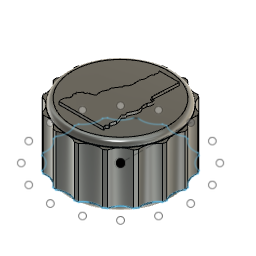
crown v4 (Autodesk Fusion 360 design; units mm, degrees)
Autodesk Fusion 360 part; units mm, degrees
note: some values were not read from the file. Set by a fixed rule: which sketch regions a step uses.
sketch "Sketch1" plane through (0, 0, 0) normal (0, 0, 1) x (1, 0, 0)
  line L0 (0, 0) -> (0, 2.54) construction
  line L1 (0, 2.54) -> (0, 3.1814)
  arc A0 (0.5741, 2.4743) -> (1.3436, 2.1555) centre (1.2174, 2.9392) ccw
  arc A1 (1.4773, 2.0662) -> (2.0662, 1.4773) centre (2.2496, 2.2496) ccw
  arc A2 (2.1555, 1.3436) -> (2.4743, 0.5741) centre (2.9392, 1.2174) ccw
  arc A3 (2.5056, 0.4165) -> (2.5056, -0.4165) centre (3.1814, 0) ccw
  arc A4 (2.4743, -0.5741) -> (2.1555, -1.3436) centre (2.9392, -1.2174) ccw
  arc A5 (2.0662, -1.4773) -> (1.4773, -2.0662) centre (2.2496, -2.2496) ccw
  arc A6 (1.3436, -2.1555) -> (0.5741, -2.4743) centre (1.2174, -2.9392) ccw
  arc A7 (-1.3436, 2.1555) -> (-0.5741, 2.4743) centre (-1.2174, 2.9392) ccw
  arc A8 (-0.4165, 2.5056) -> (0.4165, 2.5056) centre (0, 3.1814) ccw
  arc A9 (-2.0662, 1.4773) -> (-1.4773, 2.0662) centre (-2.2496, 2.2496) ccw
  arc A10 (-2.4743, 0.5741) -> (-2.1555, 1.3436) centre (-2.9392, 1.2174) ccw
  arc A11 (-2.5056, -0.4165) -> (-2.5056, 0.4165) centre (-3.1814, 0) ccw
  arc A12 (-1.4773, -2.0662) -> (-2.0662, -1.4773) centre (-2.2496, -2.2496) ccw
  arc A13 (-2.1555, -1.3436) -> (-2.4743, -0.5741) centre (-2.9392, -1.2174) ccw
  arc A14 (-0.5741, -2.4743) -> (-1.3436, -2.1555) centre (-1.2174, -2.9392) ccw
  arc A15 (0.4165, -2.5056) -> (-0.4165, -2.5056) centre (0, -3.1814) ccw
  arc A16 (-1.3436, 2.1555) -> (-1.4773, 2.0662) centre (0, 0) ccw
  arc A17 (-2.0662, 1.4773) -> (-2.1555, 1.3436) centre (0, 0) ccw
  arc A18 (-2.4743, 0.5741) -> (-2.5056, 0.4165) centre (0, 0) ccw
  arc A19 (-2.5056, -0.4165) -> (-2.4743, -0.5741) centre (0, 0) ccw
  arc A20 (-2.1555, -1.3436) -> (-2.0662, -1.4773) centre (0, 0) ccw
  arc A21 (-1.4773, -2.0662) -> (-1.3436, -2.1555) centre (0, 0) ccw
  arc A22 (-0.5741, -2.4743) -> (-0.4165, -2.5056) centre (0, 0) ccw
  arc A23 (0.4165, -2.5056) -> (0.5741, -2.4743) centre (0, 0) ccw
  arc A24 (1.3436, -2.1555) -> (1.4773, -2.0662) centre (0, 0) ccw
  arc A25 (2.0662, -1.4773) -> (2.1555, -1.3436) centre (0, 0) ccw
  arc A26 (-0.4165, 2.5056) -> (-0.5741, 2.4743) centre (0, 0) ccw
  arc A27 (0.5741, 2.4743) -> (0.4165, 2.5056) centre (0, 0) ccw
  arc A28 (1.4773, 2.0662) -> (1.3436, 2.1555) centre (0, 0) ccw
  arc A29 (2.1555, 1.3436) -> (2.0662, 1.4773) centre (0, 0) ccw
  arc A30 (2.4743, -0.5741) -> (2.5056, -0.4165) centre (0, 0) ccw
  arc A31 (2.5056, 0.4165) -> (2.4743, 0.5741) centre (0, 0) ccw
  dimension "d1" = 5.08
  dimension "d3" = 0.6413
  constraint coincident L0.start A16.centre
  constraint coincident L0.end A16
  constraint vertical L0
  constraint parallel L0 L1
  constraint coincident A8.start A16
  constraint concentric A16 A17
  constraint concentric A17 A18
  constraint concentric A18 A19
  constraint concentric A19 A20
  constraint concentric A20 A21
  constraint concentric A21 A22
  constraint concentric A22 A23
  constraint concentric A23 A24
  constraint concentric A24 A25
  constraint concentric A25 A30
  constraint coincident A0.start A30
  constraint concentric A26 A30
  constraint concentric A27 A30
  constraint concentric A28 A30
  constraint concentric A29 A30
  constraint concentric A30 A31
  measures "d1" diameter of A16
  measures "d3" distance of L0.end L1.end
extrude "Extrude1" add sketch "Sketch1" along normal blind 2.286
sketch "Sketch2" plane through (0, 0, 2.286) normal (0, 0, 1) x (-1, 0, 0)
  arc A0 (-0.5741, -2.4743) -> (-0.4165, -2.5056) centre (0, 0) ccw
  arc A1 (0.4165, -2.5056) -> (-0.4165, -2.5056) centre (0, -3.1814) ccw
  arc A2 (0.4165, -2.5056) -> (0.5741, -2.4743) centre (0, 0) ccw
  arc A3 (1.3436, -2.1555) -> (0.5741, -2.4743) centre (1.2174, -2.9392) ccw
  arc A4 (1.3436, -2.1555) -> (1.4773, -2.0662) centre (0, 0) ccw
  arc A5 (2.0662, -1.4773) -> (1.4773, -2.0662) centre (2.2496, -2.2496) ccw
  arc A6 (2.0662, -1.4773) -> (2.1555, -1.3436) centre (0, 0) ccw
  arc A7 (2.4743, -0.5741) -> (2.1555, -1.3436) centre (2.9392, -1.2174) ccw
  arc A8 (2.4743, -0.5741) -> (2.5056, -0.4165) centre (0, 0) ccw
  arc A9 (2.5056, 0.4165) -> (2.5056, -0.4165) centre (3.1814, 0) ccw
  arc A10 (2.5056, 0.4165) -> (2.4743, 0.5741) centre (0, 0) ccw
  arc A11 (2.1555, 1.3436) -> (2.4743, 0.5741) centre (2.9392, 1.2174) ccw
  arc A12 (2.1555, 1.3436) -> (2.0662, 1.4773) centre (0, 0) ccw
  arc A13 (1.4773, 2.0662) -> (2.0662, 1.4773) centre (2.2496, 2.2496) ccw
  arc A14 (1.4773, 2.0662) -> (1.3436, 2.1555) centre (0, 0) ccw
  arc A15 (0.5741, 2.4743) -> (1.3436, 2.1555) centre (1.2174, 2.9392) ccw
  arc A16 (0.5741, 2.4743) -> (0.4165, 2.5056) centre (0, 0) ccw
  arc A17 (-0.4165, 2.5056) -> (0.4165, 2.5056) centre (0, 3.1814) ccw
  arc A18 (-0.4165, 2.5056) -> (-0.5741, 2.4743) centre (0, 0) ccw
  arc A19 (-1.3436, 2.1555) -> (-0.5741, 2.4743) centre (-1.2174, 2.9392) ccw
  arc A20 (-1.3436, 2.1555) -> (-1.4773, 2.0662) centre (0, 0) ccw
  arc A21 (-2.0662, 1.4773) -> (-1.4773, 2.0662) centre (-2.2496, 2.2496) ccw
  arc A22 (-2.0662, 1.4773) -> (-2.1555, 1.3436) centre (0, 0) ccw
  arc A23 (-2.4743, 0.5741) -> (-2.1555, 1.3436) centre (-2.9392, 1.2174) ccw
  arc A24 (-2.4743, 0.5741) -> (-2.5056, 0.4165) centre (0, 0) ccw
  arc A25 (-2.5056, -0.4165) -> (-2.5056, 0.4165) centre (-3.1814, 0) ccw
  arc A26 (-2.5056, -0.4165) -> (-2.4743, -0.5741) centre (0, 0) ccw
  arc A27 (-2.1555, -1.3436) -> (-2.4743, -0.5741) centre (-2.9392, -1.2174) ccw
  arc A28 (-2.1555, -1.3436) -> (-2.0662, -1.4773) centre (0, 0) ccw
  arc A29 (-1.4773, -2.0662) -> (-2.0662, -1.4773) centre (-2.2496, -2.2496) ccw
  arc A30 (-1.4773, -2.0662) -> (-1.3436, -2.1555) centre (0, 0) ccw
  arc A31 (-0.5741, -2.4743) -> (-1.3436, -2.1555) centre (-1.2174, -2.9392) ccw
  circle A32 centre (0, 0) radius 2.3876
  constraint coincident A0.centre A2.centre
  constraint tangent A9 A32
extrude "Extrude2" add sketch "Sketch2" along normal blind 0.254 contours A32
fillet "Fillet1" radius 0.2286 1 edges at (2.226, 0.8634, 2.54)
sketch "Sketch3" plane through (0, 0, 0) normal (0, 0, -1) x (1, 0, 0)
  arc A0 (0.4165, -2.5056) -> (0.5741, -2.4743) centre (0, 0) ccw
  arc A1 (1.3436, -2.1555) -> (0.5741, -2.4743) centre (1.2174, -2.9392) ccw
  arc A2 (1.3436, -2.1555) -> (1.4773, -2.0662) centre (0, 0) ccw
  arc A3 (2.0662, -1.4773) -> (1.4773, -2.0662) centre (2.2496, -2.2496) ccw
  arc A4 (2.0662, -1.4773) -> (2.1555, -1.3436) centre (0, 0) ccw
  arc A5 (2.4743, -0.5741) -> (2.1555, -1.3436) centre (2.9392, -1.2174) ccw
  arc A6 (2.4743, -0.5741) -> (2.5056, -0.4165) centre (0, 0) ccw
  arc A7 (2.5056, 0.4165) -> (2.5056, -0.4165) centre (3.1814, 0) ccw
  arc A8 (2.5056, 0.4165) -> (2.4743, 0.5741) centre (0, 0) ccw
  arc A9 (2.1555, 1.3436) -> (2.4743, 0.5741) centre (2.9392, 1.2174) ccw
  arc A10 (2.1555, 1.3436) -> (2.0662, 1.4773) centre (0, 0) ccw
  arc A11 (1.4773, 2.0662) -> (2.0662, 1.4773) centre (2.2496, 2.2496) ccw
  arc A12 (1.4773, 2.0662) -> (1.3436, 2.1555) centre (0, 0) ccw
  arc A13 (0.5741, 2.4743) -> (1.3436, 2.1555) centre (1.2174, 2.9392) ccw
  arc A14 (0.5741, 2.4743) -> (0.4165, 2.5056) centre (0, 0) ccw
  arc A15 (-0.4165, 2.5056) -> (0.4165, 2.5056) centre (0, 3.1814) ccw
  arc A16 (-0.4165, 2.5056) -> (-0.5741, 2.4743) centre (0, 0) ccw
  arc A17 (-1.3436, 2.1555) -> (-0.5741, 2.4743) centre (-1.2174, 2.9392) ccw
  arc A18 (-1.3436, 2.1555) -> (-1.4773, 2.0662) centre (0, 0) ccw
  arc A19 (-2.0662, 1.4773) -> (-1.4773, 2.0662) centre (-2.2496, 2.2496) ccw
  arc A20 (-2.0662, 1.4773) -> (-2.1555, 1.3436) centre (0, 0) ccw
  arc A21 (-2.4743, 0.5741) -> (-2.1555, 1.3436) centre (-2.9392, 1.2174) ccw
  arc A22 (-2.4743, 0.5741) -> (-2.5056, 0.4165) centre (0, 0) ccw
  arc A23 (-2.5056, -0.4165) -> (-2.5056, 0.4165) centre (-3.1814, 0) ccw
  arc A24 (-2.5056, -0.4165) -> (-2.4743, -0.5741) centre (0, 0) ccw
  arc A25 (-2.1555, -1.3436) -> (-2.4743, -0.5741) centre (-2.9392, -1.2174) ccw
  arc A26 (-2.1555, -1.3436) -> (-2.0662, -1.4773) centre (0, 0) ccw
  arc A27 (-1.4773, -2.0662) -> (-2.0662, -1.4773) centre (-2.2496, -2.2496) ccw
  arc A28 (-1.4773, -2.0662) -> (-1.3436, -2.1555) centre (0, 0) ccw
  arc A29 (-0.5741, -2.4743) -> (-1.3436, -2.1555) centre (-1.2174, -2.9392) ccw
  arc A30 (-0.5741, -2.4743) -> (-0.4165, -2.5056) centre (0, 0) ccw
  arc A31 (0.4165, -2.5056) -> (-0.4165, -2.5056) centre (0, -3.1814) ccw
  circle A32 centre (0, 0) radius 2.3876
  constraint coincident A0.centre A2.centre
  constraint tangent A5 A32
extrude "Extrude3" add sketch "Sketch3" along normal blind 0.254 contours A32
fillet "Fillet2" radius 0.2286 1 edges at (-2.226, 0.8634, -0.254)
sketch "Sketch4" plane through (0, 0, -0.254) normal (0, 0, -1) x (1, 0, 0)
  circle A0 centre (0, 0) radius 2.159
  circle A1 centre (0, 0) radius 1.5875
  dimension "d17" = 3.175
  constraint coincident A0.centre A1.centre
  measures "d17" diameter of A1
extrude "Extrude4" cut sketch "Sketch4" against normal blind 1.27 contours A1
sketch "Sketch5" plane through (0, 0, 2.54) normal (0, 0, 1) x (-1, 0, 0)
  circle A0 centre (0, 0) radius 2.159
  line L0 (-0.8327, -1.8282) -> (0.0851, -1.8282)
  spline S0 degree 5 poles (0.0851, -1.8282) (0.0819, -1.826) (0.0755, -1.8215) (0.066, -1.814) (0.0539, -1.8027) (0.0396, -1.7866) (0.0263, -1.7686) (0.0147, -1.7493) (0.0058, -1.7292) (0.0007, -1.7096) (0.0007, -1.6913) (0.0061, -1.6751) (0.0162, -1.661) (0.0284, -1.6482) (0.0394, -1.6351) (0.0457, -1.6205) (0.0454, -1.6035) (0.0387, -1.5849) (0.0292, -1.5667) (0.0213, -1.5514) (0.0193, -1.5408) (0.0259, -1.535) (0.0401, -1.531) (0.0583, -1.524) (0.0761, -1.5088) (0.0893, -1.4814) (0.0956, -1.4407) (0.0955, -1.3893) (0.0912, -1.3318) (0.086, -1.2741) (0.083, -1.2217) (0.0849, -1.179) (0.0927, -1.1472) (0.1052, -1.1244) (0.12, -1.1066) (0.1344, -1.089) (0.1459, -1.0671) (0.153, -1.0381) (0.1556, -1.0012) (0.1546, -0.9571) (0.1513, -0.9076) (0.1474, -0.8549) (0.1445, -0.8014) (0.1438, -0.749) (0.1459, -0.6991) (0.1511, -0.6527) (0.1597, -0.6107) (0.1715, -0.5734) (0.1866, -0.5414) (0.2048, -0.5147) (0.2261, -0.4936) (0.2456, -0.4811) (0.2617, -0.4742) (0.273, -0.4707) (0.2788, -0.4693) knots 0 0 0 0 0 0 0.02 0.04 0.06 0.08 0.1 0.12 0.14 0.16 0.18 0.2 0.22 0.24 0.26 0.28 0.3 0.32 0.34 0.36 0.38 0.4 0.42 0.44 0.46 0.48 0.5 0.52 0.54 0.56 0.58 0.6 0.62 0.64 0.66 0.68 0.7 0.72 0.74 0.76 0.78 0.8 0.82 0.84 0.86 0.88 0.9 0.92 0.94 0.96 0.98 1 1 1 1 1 1
  line L1 (0.2788, -0.4693) -> (0.2788, -0.372)
  line L2 (0.2788, -0.372) -> (0.4906, -0.0512)
  spline S1 degree 5 poles (0.4906, -0.0512) (0.4887, -0.0439) (0.4852, -0.0295) (0.4811, -0.0088) (0.4778, 0.0169) (0.4774, 0.0462) (0.4804, 0.0728) (0.4867, 0.097) (0.4959, 0.1195) (0.5074, 0.1412) (0.5203, 0.1634) (0.5337, 0.1872) (0.5466, 0.2136) (0.5582, 0.2433) (0.5675, 0.276) (0.5738, 0.3111) (0.5766, 0.3473) (0.5758, 0.3833) (0.5717, 0.4175) (0.565, 0.4489) (0.557, 0.4767) (0.5497, 0.5008) (0.5451, 0.5214) (0.5447, 0.539) (0.5501, 0.5542) (0.5617, 0.5679) (0.579, 0.5806) (0.6013, 0.5928) (0.6272, 0.6049) (0.6552, 0.6166) (0.6838, 0.6271) (0.7116, 0.6353) (0.7375, 0.6404) (0.7605, 0.642) (0.78, 0.6405) (0.7956, 0.6381) (0.8075, 0.6378) (0.8162, 0.6428) (0.8227, 0.655) (0.8285, 0.674) (0.8354, 0.6966) (0.8451, 0.7182) (0.859, 0.7345) (0.8775, 0.7427) (0.8998, 0.7429) (0.9239, 0.7386) (0.9471, 0.7348) (0.9671, 0.7361) (0.9826, 0.7459) (0.9938, 0.764) (1.0026, 0.7873) (1.0113, 0.8114) (1.0223, 0.8318) (1.0369, 0.8459) (1.0546, 0.8539) (1.0734, 0.8587) (1.0907, 0.8641) (1.1037, 0.8733) (1.1102, 0.8878) (1.1094, 0.9054) (1.1016, 0.9227) (1.0882, 0.936) (1.0717, 0.9427) (1.0557, 0.9434) (1.0441, 0.941) (1.0402, 0.9394) (1.0458, 0.9422) (1.0597, 0.9507) (1.0782, 0.9644) (1.0966, 0.9817) (1.1102, 1.0005) (1.1157, 1.0193) (1.1125, 1.0379) (1.1019, 1.0571) (1.0869, 1.0781) (1.0706, 1.102) (1.0562, 1.1292) (1.0458, 1.1588) (1.0406, 1.1894) (1.041, 1.219) (1.047, 1.246) (1.0577, 1.2693) (1.0722, 1.2891) (1.0891, 1.3065) (1.1069, 1.3233) (1.1241, 1.3417) (1.1394, 1.3638) (1.1517, 1.3914) (1.1604, 1.4256) (1.1649, 1.4673) (1.165, 1.5169) (1.1613, 1.5631) (1.1564, 1.6014) (1.1523, 1.6287) (1.15, 1.6427) knots 0 0 0 0 0 0 0.01111111 0.02222222 0.03333333 0.04444444 0.05555556 0.06666667 0.07777778 0.08888889 0.1 0.11111111 0.12222222 0.13333333 0.14444444 0.15555556 0.16666667 0.17777778 0.18888889 0.2 0.21111111 0.22222222 0.23333333 0.24444444 0.25555556 0.26666667 0.27777778 0.28888889 0.3 0.31111111 0.32222222 0.33333333 0.34444444 0.35555556 0.36666667 0.37777778 0.38888889 0.4 0.41111111 0.42222222 0.43333333 0.44444444 0.45555556 0.46666667 0.47777778 0.48888889 0.5 0.51111111 0.52222222 0.53333333 0.54444444 0.55555556 0.56666667 0.57777778 0.58888889 0.6 0.61111111 0.62222222 0.63333333 0.64444444 0.65555556 0.66666667 0.67777778 0.68888889 0.7 0.71111111 0.72222222 0.73333333 0.74444444 0.75555556 0.76666667 0.77777778 0.78888889 0.8 0.81111111 0.82222222 0.83333333 0.84444444 0.85555556 0.86666667 0.87777778 0.88888889 0.9 0.91111111 0.92222222 0.93333333 0.94444444 0.95555556 0.96666667 0.97777778 0.98888889 1 1 1 1 1 1
  line L3 (1.15, 1.6427) -> (-0.8756, 1.6427)
  line L4 (-0.8756, 1.6427) -> (-0.8331, 1.5362)
  line L5 (-0.8331, 1.5362) -> (-0.9219, 1.4397)
  line L6 (-0.8327, -1.8282) -> (-0.7756, -0.6654)
  line L7 (-0.9219, 1.4397) -> (-0.8544, 1.3435)
  line L8 (-0.8544, 1.3435) -> (-0.9219, 1.1069)
  spline S2 degree 5 poles (-0.9219, 1.1069) (-0.9218, 1.1038) (-0.9213, 1.097) (-0.9197, 1.0853) (-0.9161, 1.0667) (-0.909, 1.0385) (-0.8994, 1.0058) (-0.8876, 0.9694) (-0.874, 0.9308) (-0.8591, 0.8922) (-0.8439, 0.856) (-0.8292, 0.8245) (-0.8163, 0.7991) (-0.8066, 0.7801) (-0.8018, 0.7662) (-0.8031, 0.7548) (-0.8114, 0.7434) (-0.8262, 0.7296) (-0.8453, 0.7129) (-0.8649, 0.6941) (-0.8809, 0.6749) (-0.8896, 0.6572) (-0.8891, 0.642) (-0.8804, 0.6292) (-0.8667, 0.6173) (-0.8523, 0.6044) (-0.8417, 0.5883) (-0.8378, 0.5676) (-0.8418, 0.5415) (-0.8531, 0.5103) (-0.8702, 0.4746) (-0.891, 0.4351) (-0.9132, 0.3928) (-0.935, 0.3487) (-0.9546, 0.3033) (-0.9708, 0.2575) (-0.9824, 0.2116) (-0.9886, 0.1661) (-0.9887, 0.1214) (-0.9824, 0.0776) (-0.9695, 0.0349) (-0.9539, 0.0015) (-0.9391, -0.023) (-0.9279, -0.0391) (-0.9219, -0.0471) knots 0 0 0 0 0 0 0.025 0.05 0.075 0.1 0.125 0.15 0.175 0.2 0.225 0.25 0.275 0.3 0.325 0.35 0.375 0.4 0.425 0.45 0.475 0.5 0.525 0.55 0.575 0.6 0.625 0.65 0.675 0.7 0.725 0.75 0.775 0.8 0.825 0.85 0.875 0.9 0.925 0.95 0.975 1 1 1 1 1 1
  line L9 (-0.9219, -0.0471) -> (-0.9219, -0.2774)
  spline S3 degree 5 poles (-0.7756, -0.6654) (-0.7751, -0.6632) (-0.7742, -0.6588) (-0.7736, -0.6522) (-0.7744, -0.6434) (-0.7778, -0.6322) (-0.7836, -0.6209) (-0.7916, -0.6095) (-0.8011, -0.5978) (-0.8115, -0.5859) (-0.8218, -0.5736) (-0.831, -0.561) (-0.8386, -0.5481) (-0.8442, -0.5351) (-0.8482, -0.5225) (-0.8513, -0.5106) (-0.8544, -0.5001) (-0.8585, -0.4913) (-0.8644, -0.4848) (-0.8728, -0.4807) (-0.8838, -0.4792) (-0.8949, -0.48) (-0.9044, -0.4818) (-0.9113, -0.4835) (-0.9149, -0.4844) knots 0 0 0 0 0 0 0.05 0.1 0.15 0.2 0.25 0.3 0.35 0.4 0.45 0.5 0.55 0.6 0.65 0.7 0.75 0.8 0.85 0.9 0.95 1 1 1 1 1 1
  line L10 (-0.9149, -0.4844) -> (-0.9149, -0.5641)
  spline S4 degree 5 poles (-0.9219, -0.2774) (-0.9242, -0.279) (-0.9286, -0.2826) (-0.9352, -0.2893) (-0.9435, -0.3009) (-0.9533, -0.32) (-0.9624, -0.3435) (-0.9705, -0.371) (-0.9774, -0.4017) (-0.9827, -0.4341) (-0.9858, -0.4664) (-0.9862, -0.4967) (-0.9834, -0.5231) (-0.9772, -0.5442) (-0.9673, -0.5592) (-0.9537, -0.5678) (-0.94, -0.5695) (-0.9281, -0.5679) (-0.9194, -0.5656) (-0.9149, -0.5641) knots 0 0 0 0 0 0 0.066667 0.133333 0.2 0.266667 0.333333 0.4 0.466667 0.533333 0.6 0.666667 0.733333 0.8 0.866667 0.933333 1 1 1 1 1 1
  point P0 (0.0188, -1.7555)
  point P1 (0.0092, -1.672)
  point P2 (0.0445, -1.6078)
  point P3 (0.0221, -1.5405)
  point P4 (0.0851, -1.4859)
  point P5 (0.0851, -1.1939)
  point P6 (0.1408, -1.0751)
  point P7 (0.1472, -0.8473)
  point P8 (0.1716, -0.5765)
  point P9 (0.4906, 0.1055)
  point P10 (0.5536, 0.2327)
  point P11 (0.5688, 0.4295)
  point P12 (0.5476, 0.5445)
  point P13 (0.6354, 0.6081)
  point P14 (0.7695, 0.641)
  point P15 (0.821, 0.6531)
  point P16 (0.8694, 0.7379)
  point P17 (0.9724, 0.7409)
  point P18 (1.0269, 0.8348)
  point P19 (1.1012, 0.8735)
  point P20 (1.0823, 0.9374)
  point P21 (1.0437, 0.9412)
  point P22 (1.1094, 1.003)
  point P23 (1.0708, 1.1033)
  point P24 (1.0515, 1.2539)
  point P25 (1.1305, 1.352)
  point P26 (-0.8881, 0.9717)
  point P27 (-0.8157, 0.7979)
  point P28 (-0.8205, 0.7351)
  point P29 (-0.8881, 0.6531)
  point P30 (-0.8447, 0.5903)
  point P31 (-0.8881, 0.4406)
  point P32 (-0.9847, 0.1895)
  point P33 (-0.7918, -0.6096)
  point P34 (-0.8384, -0.5476)
  point P35 (-0.8591, -0.4917)
  point P36 (-0.9701, -0.3713)
  point P37 (-0.9821, -0.5241)
  constraint horizontal L0
  constraint vertical L1
  constraint horizontal L3
  constraint vertical L9
  constraint vertical L10
extrude "Extrude5" add sketch "Sketch5" along normal blind 0.127 contours L0 S0 L1 L2 S1 L3 L4 L5 L6 L7 L8 S2 L9 S3 L10 S4
equation "d3 = ( 1 / 32 ) * 1 in - 0.006 in"
